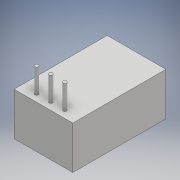
# Autodesk Inventor part: Circuit_OKI-78SR
Saved by Autodesk Inventor 2018 (Build 220112000, 112)
## iProperties
Created: 2018-02-15
Part Number: Circuit_OKI-78SR
Material: 一般
Document SubType Name: Modeling
Designer: sktom
Density: 1 g/cm^3
Appearance: 既定
Author: sktom
Autodesk Inventor part; units mm, degrees
ref_plane "YZ Plane" through (0, 0, 0) normal (1, 0, 0) x (0, 1, 0)
ref_plane "XZ Plane" through (0, 0, 0) normal (0, 1, 0) x (-1, 0, 0)
ref_plane "XY Plane" through (0, 0, 0) normal (0, 0, 1) x (1, 0, 0)
sketch "スケッチ1" plane through (0, 0, 0) normal (0, 0, 1) x (1, 0, 0)
  line L0 (-5.2, -8.25) -> (5.2, -8.25)
  line L1 (5.2, -8.25) -> (5.2, 8.25)
  line L2 (5.2, 8.25) -> (-5.2, 8.25)
  line L3 (-5.2, 8.25) -> (-5.2, -8.25)
  line L4 (-5.2, -8.25) -> (5.2, 8.25) construction
  line L5 (5.2, -8.25) -> (-5.2, 8.25) construction
  point P0 (0, 0)
  dimension "d0" = 10.4
  dimension "d1" = 16.5
  constraints: 12 end point, 2 midpoint, 2 parallel, 1 horizontal, 1 perpendicular
  measures "d0" distance of L1.end L2.end
  measures "d1" distance of L0.end L1.end
extrude "押し出し1" add sketch "スケッチ1" along normal blind 7.6
sketch "スケッチ2" plane through (0, 0, 7.6) normal (0, 0, 1) x (1, 0, 0)
  circle A0 centre (0, -6.95) radius 0.3175
  circle A1 centre (2.5, -6.95) radius 0.3175
  circle A2 centre (-2.5, -6.95) radius 0.3175
  line L0 (-5.2, -8.25) -> (5.2, -8.25) projected
  point P0 (0, 0)
  dimension "d4" = 1.3
  dimension "d5" = 0.635
  dimension "d6" = 2.5
  dimension "d7" = 2.5
  constraints: 3 centre point, 2 equal radius, 2 horizontal alignment, 1 vertical alignment
  measures "d4" distance from line of L0 A0.centre
  measures "d5" diameter of A0
  measures "d6" distance of A0.centre A1.centre
  measures "d7" distance of A2.centre A0.centre
extrude "押し出し2" add sketch "スケッチ2" along normal blind 4.3
